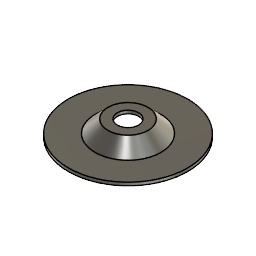
avo_vcm_mk3_knob_skirt (Autodesk Fusion 360 design; units mm, degrees)
Autodesk Fusion 360 part; units mm, degrees
sketch "Sketch1" plane through (0, 0, 0) normal (1, 0, 0) x (0, 1, 0)
  line L0 (-31.75, 0) -> (31.75, 0) construction
  line L1 (-31.75, 0) -> (-31.75, 1.7)
  line L2 (31.75, 0) -> (31.75, 1.7)
  line L3 (0, 0) -> (0, 8.4) construction
  line L4 (-5.65, 8.4) -> (5.65, 8.4) construction
  line L5 (-10.65, 8.4) -> (10.65, 8.4) construction
  line L6 (-5.65, 8.4) -> (-10.65, 8.4)
  line L7 (5.65, 8.4) -> (10.65, 8.4)
  line L8 (-17.5, 1.7) -> (17.5, 1.7) construction
  line L9 (-31.75, 1.7) -> (-17.5, 1.7)
  line L10 (-17.5, 1.7) -> (-10.65, 8.4)
  line L11 (31.75, 1.7) -> (17.5, 1.7)
  line L12 (17.5, 1.7) -> (10.65, 8.4)
  line L13 (-30.05, 0) -> (-16.8068, 0)
  line L14 (-16.8068, 0) -> (-9.9568, 6.7)
  line L15 (-5.65, 6.7) -> (-9.9568, 6.7)
  line L16 (30.05, 0) -> (16.8068, 0)
  line L17 (16.8068, 0) -> (9.9568, 6.7)
  line L18 (5.65, 6.7) -> (9.9568, 6.7)
  line L19 (-5.65, 6.7) -> (-5.65, 8.4)
  line L20 (5.65, 6.7) -> (5.65, 8.4)
  line L21 (-30.05, 0) -> (-31.75, 0)
  line L22 (30.05, 0) -> (31.75, 0)
  dimension "d1" = 63.5
  dimension "d2" = 1.7
  dimension "d3" = 1.7
  dimension "d4" = 8.4
  dimension "d5" = 11.3
  dimension "d6" = 21.3
  dimension "d7" = 5
  dimension "d8" = 5
  dimension "d9" = 35
  dimension "d10" = 1.7
  dimension "d11" = -1.7
  constraint horizontal L0
  constraint midpoint L3.start L0
  constraint perpendicular L0 L1
  constraint perpendicular L0 L2
  constraint coincident L3.start origin
  constraint perpendicular L0 L3
  constraint horizontal L4
  constraint midpoint L3.end L4
  constraint horizontal L5
  constraint midpoint L3.end L5
  constraint horizontal L8
  constraint perpendicular L1 L9
  constraint perpendicular L5 L19
  constraint perpendicular L5 L20
  constraint perpendicular L1 L21
  constraint perpendicular L2 L22
  measures "d1" distance of L0.start L0.end
  measures "d2" distance of L0.start L1.end
  measures "d3" distance of L0.end L2.end
  measures "d4" distance of L3.start L3.end
  measures "d5" distance of L4.start L4.end
  measures "d6" distance of L5.start L5.end
  measures "d7" distance of L4.start L5.start
  measures "d8" distance of L4.end L5.end
  measures "d9" distance of L8.start L8.end
revolve "Revolve1" add sketch "Sketch1" angle 360 about axis through (0, 0, 0) along (0, 0, 1) contours L1 L6 L9 L10 L13 L14 L15 L19 L21
sketch "Sketch2" plane through (0, 0, 0) normal (0, 0, -1) x (1, 0, 0)
  circle A0 centre (0, 0) radius 16.8068
  circle A1 centre (0, 0) radius 31.75
  line L0 (0.5, -31.75) -> (-0.5, -31.75)
  line L1 (-0.5, -31.75) -> (-0.5, -23.25)
  line L2 (-0.5, -23.25) -> (0.5, -23.25)
  line L3 (0.5, -23.25) -> (0.5, -31.75)
  circle A2 centre (0, 0) radius 31.75
  line L4 (0, -31.75) -> (0, 31.75) construction
  dimension "d13" = 1
  dimension "d14" = 8.5
  dimension "d15" = 63.5
  constraint horizontal L0
  constraint vertical L1
  constraint horizontal L2
  constraint vertical L3
  constraint vertical L4
  constraint midpoint A0.centre L4
  constraint midpoint L0 L4.start
  measures "d13" distance of L0.start L0.end
  measures "d14" distance of L0.start L2.end
  measures "d15" distance of L4.start L4.end
extrude "Extrude1" cut sketch "Sketch2" against normal blind 0.4 contours A1 L1 L2 L3 A2 picked at (0, -26.0833)
